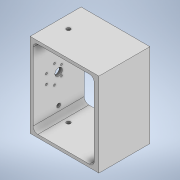
# Autodesk Inventor part: caja conexion
Saved by Autodesk Inventor 2020.3 (Build 243373000, 373)
## iProperties
Created: 2021-02-11
Part Number: caja conexion
Material: Generic
Document SubType Name: Modeling
Designer: Yu Jinyu
Density: 1 g/cm^3
Appearance: Default
Author: Yu Jinyu
Autodesk Inventor part; units mm, degrees
ref_plane "YZ Plane" through (0, 0, 0) normal (1, 0, 0) x (0, 1, 0)
ref_plane "XZ Plane" through (0, 0, 0) normal (0, 1, 0) x (-1, 0, 0)
ref_plane "XY Plane" through (0, 0, 0) normal (0, 0, 1) x (1, 0, 0)
sketch "Sketch1" plane through (0, 0, 0) normal (0, 0, 1) x (1, 0, 0)
  line L0 (-50.984, -65) -> (50.984, -65)
  line L1 (50.984, -65) -> (50.984, 65)
  line L2 (50.984, 65) -> (-50.984, 65)
  line L3 (-50.984, 65) -> (-50.984, -65)
  line L4 (-50.984, -65) -> (50.984, 65) construction
  line L5 (50.984, -65) -> (-50.984, 65) construction
  line L6 (-55.984, 70) -> (55.984, 70)
  line L7 (55.984, 70) -> (55.984, -70)
  line L8 (55.984, -70) -> (-55.984, -70)
  line L9 (-55.984, -70) -> (-55.984, 70)
  point P0 (0, 0)
  dimension "d0" = 101.968
  dimension "d1" = 130
  dimension "d2" = 5
  constraints: 20 end point, 4 parallel, 2 midpoint, 2 perpendicular, 1 horizontal, 3 other
  measures "d0" distance of L2.end L1.end
  measures "d1" distance of L1.end L0.end
  measures "d2" distance between parallel lines of L2 L6
extrude "Extrusion1" add sketch "Sketch1" along normal blind 50
sketch "Sketch5" plane through (50.984, -65, 0) normal (-1, 0, 0) x (0, 0, 1)
  line L0 (0, -5) -> (50, -5) projected
  line L1 (0, 135) -> (50, 135) projected
  circle A0 centre (25, 65) radius 12
  line L2 (50, 135) -> (50, -5) projected
  point P0 (0, 65)
  dimension "d14" = 140
  dimension "d15" = 24
  dimension "d16" = 25
  dimension "d17" = 70
  constraints: 1 centre point
  measures "d14" distance between parallel lines of L0 L1
  measures "d15" diameter of A0
  measures "d16" distance from line of A0.centre L2
  measures "d17" distance from line of L1 A0.centre
extrude "Extrusion5" cut sketch "Sketch5" against normal blind 2.778
sketch "Sketch6" plane through (55.984, -70, 0) normal (1, 0, 0) x (0, 0, -1)
  line L0 (0, 0) -> (0, 140) projected
  line L1 (0, 140) -> (-50, 140) projected
  line L2 (-50, 0) -> (-50, 140) projected
  line L3 (0, 0) -> (-50, 0) projected
  point P0 (0, 70)
extrude "Extrusion6" add sketch "Sketch6" along normal blind 2.778
sketch "Sketch8" plane through (0, 0, 0) normal (0, 0, -1) x (-1, 0, 0)
  line L0 (55.984, -70) -> (-58.762, -70) projected
  line L1 (55.984, 70) -> (55.984, -70) projected
  line L2 (55.984, 70) -> (-58.762, 70) projected
  line L3 (-58.762, -70) -> (-58.762, 70) projected
  line L4 (50.984, -65) -> (50.984, 65) projected
  line L5 (-50.984, -65) -> (50.984, -65) projected
  line L6 (-50.984, 65) -> (-50.984, -65) projected
  line L7 (50.984, 65) -> (-50.984, 65) projected
  point P0 (0, 0)
extrude "Extrusion8" add sketch "Sketch8" along normal blind 17.5
sketch "Sketch9" plane through (0, 0, 50) normal (0, 0, 1) x (1, 0, 0)
  line L0 (-55.984, -70) -> (58.762, -70) projected
  line L1 (58.762, 70) -> (58.762, -70) projected
  line L2 (-55.984, 70) -> (58.762, 70) projected
  line L3 (-55.984, 70) -> (-55.984, -70) projected
  line L4 (-50.984, -65) -> (-50.984, 65) projected
  line L5 (-50.984, 65) -> (50.984, 65) projected
  line L6 (50.984, 65) -> (50.984, -65) projected
  line L7 (50.984, -65) -> (-50.984, -65) projected
  point P0 (0, 0)
extrude "Extrusion9" add sketch "Sketch9" along normal blind 17.5
fillet "Fillet1" radius 8 1 edges at (-50.984, -65, 25)
fillet "Fillet2" radius 8 3 edges at (50.984, -65, 25) (50.984, 65, 25) (-50.984, 65, 25)
sketch "Sketch10" plane through (-55.984, -70, -17.5) normal (-1, 0, 0) x (0, 0, 1)
  circle A0 centre (42.5, 70) radius 6.25
  circle A1 centre (37.767, 78.237) radius 1.65
  line L0 (0, 0) -> (0, 140) projected
  line L1 (85, 0) -> (0, 0) projected
  circle A2 centre (37.733, 61.7537) radius 1.65
  circle A3 centre (49.5, 85.5) radius 1.65
  circle A4 centre (49.5, 54.5) radius 1.65
  circle A5 centre (62.923, 77.75) radius 1.65
  circle A6 centre (62.923, 62.25) radius 1.65
  point P0 (17.5, 70)
  dimension "d31" = 12.5
  dimension "d32" = 3.3
  dimension "d33" = 37.767
  dimension "d34" = 78.237
  dimension "d35" = 3.3
  dimension "d36" = 37.733
  dimension "d38" = 61.7537
  dimension "d39" = 3.3
  dimension "d41" = 85.5
  dimension "d42" = 49.5
  dimension "d43" = 3.3
  dimension "d44" = 54.5
  dimension "d45" = 3.3
  dimension "d46" = 77.75
  dimension "d47" = 62.923
  dimension "d48" = 3.3
  dimension "d49" = 62.25
  dimension "d50" = 62.923
  constraints: 7 centre point, 1 coincident
  measures "d31" diameter of A0
  measures "d32" diameter of A1
  measures "d33" distance from line of A1.centre L0
  measures "d34" distance from line of A1.centre L1
  measures "d35" diameter of A2
  measures "d36" distance from line of L0 A2.centre
  measures "d38" distance from line of L1 A2.centre
  measures "d39" diameter of A3
  measures "d41" distance from line of A3.centre L1
  measures "d42" distance from line of L0 A3.centre
  measures "d43" diameter of A4
  measures "d44" distance from line of A4.centre L1
  measures "d45" diameter of A5
  measures "d46" distance from line of A5.centre L1
  measures "d47" distance from line of L0 A5.centre
  measures "d48" diameter of A6
  measures "d49" distance from line of A6.centre L1
  measures "d50" distance from line of L0 A6.centre
extrude "Extrusion10" cut sketch "Sketch10" against normal blind 5
sketch "Sketch11" plane through (-55.984, -70, -17.5) normal (-1, 0, 0) x (0, 0, 1)
  circle A0 centre (42.5, 21.5) radius 3.25
  circle A1 centre (42.5, 118.5) radius 3.25
  line L0 (0, 140) -> (85, 140) projected
  line L1 (85, 0) -> (0, 0) projected
  point P0 (17.5, 70)
  dimension "d53" = 6.5
  dimension "d54" = 6.5
  dimension "d58" = 21.5
  dimension "d59" = 21.5
  constraints: 2 centre point
  measures "d53" diameter of A0
  measures "d54" diameter of A1
  measures "d58" distance from line of L0 A1.centre
  measures "d59" distance from line of L1 A0.centre
extrude "Extrusion12" cut sketch "Sketch11" against normal blind 10
sketch "Sketch12" plane through (-55.984, -70, -17.5) normal (0, -1, 0) x (1, 0, 0)
  circle A0 centre (21.5, 42.5) radius 3.25
  line L0 (0, 85) -> (0, 0) projected
  point P0 (55.984, 17.5)
  dimension "d62" = 6.5
  dimension "d63" = 21.5
  constraints: 1 centre point
  measures "d62" diameter of A0
  measures "d63" distance from line of L0 A0.centre
sketch "Sketch13" plane through (-55.984, 70, -17.5) normal (0, 1, 0) x (1, 0, 0)
  circle A0 centre (21.5, -42.5) radius 3.25
  line L0 (0, 0) -> (0, -85) projected
  point P0 (55.984, -17.5)
  dimension "d66" = 6.5
  dimension "d67" = 21.5
  constraints: 1 centre point
  measures "d66" diameter of A0
  measures "d67" distance from line of L0 A0.centre
extrude "Extrusion13" cut sketch "Sketch12" against normal blind 10
extrude "Extrusion14" cut sketch "Sketch13" against normal blind 10
body "Solid1"
